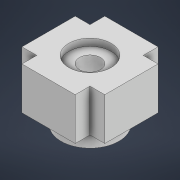
# Autodesk Inventor part: Zahnrad_innen_mitte
Saved by Autodesk Inventor 2021 (Build 250183000, 183)
## iProperties
Created: 2021-01-01
Part Number: Zahnrad_innen_mitte
Material: Generisch
Document SubType Name: Modeling
Designer: laure
Density: 1 g/cm^3
Appearance: Vorgabe
Author: laure
## iProperties of the stored document _3D-Druck.ipt
Created: 2021-01-01
Part Number: _3D-Druck
Material: Generisch
Document SubType Name: Modeling
Designer: laure
Density: 1 g/cm^3
Appearance: Vorgabe
Author: laure
Autodesk Inventor part; units mm, degrees
ref_plane "YZ Plane" through (0, 0, 0) normal (1, 0, 0) x (0, 1, 0)
ref_plane "XZ Plane" through (0, 0, 0) normal (0, 1, 0) x (-1, 0, 0)
ref_plane "XY Plane" through (0, 0, 0) normal (0, 0, 1) x (1, 0, 0)
sketch "Skizze1" plane through (0, 0, 0) normal (0, 1, 0) x (-1, 0, 0)
  circle A0 centre (0, 0) radius 3.5
  line L0 (5.875, -5.875) -> (-5.875, -5.875)
  line L1 (-5.875, -5.875) -> (-5.875, 5.875)
  line L2 (-5.875, 5.875) -> (5.875, 5.875)
  line L3 (5.875, 5.875) -> (5.875, -5.875)
  line L4 (8.225, 0) -> (-8.225, 0) projected
  line L5 (0.75, 5.875) -> (-0.75, 5.875)
  line L6 (0, -8.225) -> (0, 8.225) projected
  point P0 (0.75, -5.875)
  point P1 (-5.875, -0.75)
  point P2 (5.875, -0.75)
  dimension "d1" = 7
  dimension "d2" = 11.75
  dimension "d3" = 11.75
  constraints: 10 end point, 4 point on line, 2 horizontal, 2 parallel, 1 centre point, 1 perpendicular, 2 other
  measures "d1" diameter of A0
  measures "d2" distance between parallel lines of L3 L1
  measures "d3" distance between parallel lines of L2 L0
extrude "Extrusion1" add sketch "Skizze1" along normal mid plane 6
sketch "Skizze2" plane through (0, 3, 0) normal (0, 1, 0) x (1, 0, 0)
  circle A0 centre (0, 0) radius 3
  dimension "d14" = 6
  constraints: 1 centre point, 1 coincident
  measures "d14" diameter of A0
ref_plane "Arbeitsebene1" through (0, -0.5, 0) normal (0, 1, 0) x (1, 0, 0)
sketch "Skizze4" plane through (0, -3, 0) normal (0, -1, 0) x (1, 0, 0)
  circle A0 centre (0, 0) radius 2.85
  circle A1 centre (0, 0) radius 1.4 projected
  circle A2 centre (0, 0) radius 4.1
  dimension "d20" = 5.7
  dimension "d21" = 8.2
  constraints: 2 centre point, 2 coincident
  measures "d20" diameter of A0
  measures "d21" diameter of A2
extrude "Extrusion4" add sketch "Skizze4" along normal blind 2.5 contours A2
sketch "Skizze5" plane through (0, 3, 0) normal (0, 1, 0) x (1, 0, 0)
  line L0 (-5.875, 5.875) -> (5.875, 5.875) projected
  line L1 (-5.875, 5.875) -> (-3.775, 5.875)
  line L2 (-3.775, 5.875) -> (-3.775, 3.775)
  line L3 (-3.775, 3.775) -> (-5.875, 3.775)
  line L4 (-5.875, 3.775) -> (-5.875, 5.875)
  line L5 (-5.875, 5.875) -> (5.875, 5.875) projected
  line L6 (5.875, 5.875) -> (3.775, 5.875)
  line L7 (3.775, 5.875) -> (3.775, 3.775)
  line L8 (3.775, 3.775) -> (5.875, 3.775)
  line L9 (5.875, 3.775) -> (5.875, 5.875)
  line L10 (-5.875, -5.875) -> (-5.875, 5.875) projected
  line L11 (-5.875, -5.875) -> (-3.775, -5.875)
  line L12 (-3.775, -5.875) -> (-3.775, -3.775)
  line L13 (-3.775, -3.775) -> (-5.875, -3.775)
  line L14 (-5.875, -3.775) -> (-5.875, -5.875)
  line L15 (5.875, -5.875) -> (-5.875, -5.875) projected
  line L16 (5.875, -5.875) -> (3.775, -5.875)
  line L17 (3.775, -5.875) -> (3.775, -3.775)
  line L18 (3.775, -3.775) -> (5.875, -3.775)
  line L19 (5.875, -3.775) -> (5.875, -5.875)
  point P0 (0, 0)
  point P1 (-0.75, 5.75)
  point P2 (0.75, 5.75)
  point P3 (-5.75, -0.75)
  point P4 (0.75, -5.75)
  dimension "d24" = 2.1
  dimension "d25" = 2.1
  dimension "d26" = 2.1
  dimension "d27" = 2.1
  dimension "d28" = 2.1
  dimension "d29" = 2.1
  dimension "d30" = 2.1
  dimension "d31" = 2.1
  constraints: 32 end point, 8 parallel, 4 horizontal, 4 perpendicular, 4 other
  measures "d24" distance of L2.end L3.end
  measures "d25" distance of L1.end L2.end
  measures "d26" distance of L8.end L7.end
  measures "d27" length of L8
  measures "d28" distance of L13.end L12.end
  measures "d29" distance of L12.end L11.end
  measures "d30" distance of L17.end L18.end
  measures "d31" distance of L16.end L17.end
extrude "Extrusion5" cut sketch "Skizze5" against normal blind 6
extrude "Extrusion6" cut sketch "Skizze2" against normal blind 1
sketch "Skizze6" plane through (0, 2, 0) normal (0, 1, 0) x (1, 0, 0)
  circle A0 centre (0, 0) radius 1.5
  dimension "d38" = 3
  constraints: 1 centre point, 1 coincident
  measures "d38" diameter of A0
extrude "Extrusion7" cut sketch "Skizze6" against normal up to surface (5 mm away)
